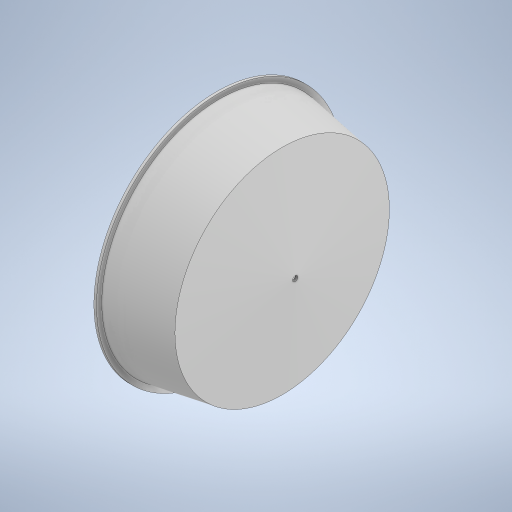
# Autodesk Inventor part: kab
Saved by Autodesk Inventor 2023.2 (Build 272271000, 271)
## iProperties
Created: 2023-03-22
Part Number: kab
Material: Generic
Document SubType Name: Modeling
Designer: sarp1
Density: 1 g/cm^3
Appearance: Default
Author: sarp1
Autodesk Inventor part; units mm, degrees
ref_plane "YZ Plane" through (0, 0, 0) normal (1, 0, 0) x (0, 1, 0)
ref_plane "XZ Plane" through (0, 0, 0) normal (0, 1, 0) x (-1, 0, 0)
ref_plane "XY Plane" through (0, 0, 0) normal (0, 0, 1) x (1, 0, 0)
sketch "Sketch1" plane through (0, 0, 0) normal (0, 0, 1) x (1, 0, 0)
  line L0 (13.5963, 0) -> (13.5963, -0.5)
  line L1 (13.5963, -0.5) -> (0, -0.5)
  line L2 (13, 0) -> (13.5963, 0)
  line L3 (-5.5, 23.9002) -> (9.5, 23.9002)
  line L4 (-5.5, 20) -> (-5.5, 22)
  line L5 (-5.5, 22) -> (-5, 22)
  line L6 (-5.5, 22) -> (-5, 22)
  line L7 (-5, 22) -> (-5, 23)
  line L8 (-5, 23) -> (-5.5, 23)
  line L9 (-5.5, 23) -> (-5.5, 22)
  line L10 (13.5963, 0) -> (13.5963, 20)
  line L11 (8.1189, -3.8338) -> (31.713, -3.8338) construction
  line L12 (-5.5, 20) -> (6.5, 20)
  line L13 (9.5, 0) -> (9, 0)
  line L14 (9, 0) -> (6.5, 20)
  line L15 (6.5, 20) -> (7, 20)
  line L16 (7, 20) -> (9.5, 0)
  line L17 (-5, 22) -> (7, 20)
  dimension "d7" = 15
  dimension "d11" = 2
  dimension "d12" = 0.5
  dimension "d13" = 1
  dimension "d17" = 20
  dimension "d19" = 12
  dimension "d20" = 0.5
  dimension "d21" = 0.5
  constraints: 36 end point, 5 horizontal, 3 perpendicular, 3 vertical, 2 parallel, 1 point on line
  measures "d7" distance of L3.start L3.end
  measures "d11" distance of L4.start L4.end
  measures "d12" distance of L4.end L5.end
  measures "d13" distance of L7.end L6.end
  measures "d17" distance of L0.start L10.end
  measures "d19" distance of L4.start L12.end
  measures "d20" distance of L13.start L13.end
  measures "d21" distance of L12.end L15.end
revolve "Revolution1" add sketch "Sketch1" angle 360 about axis through (13.5963, -0.5, 0) along (-1, 0, 0)
body "Solid1"
